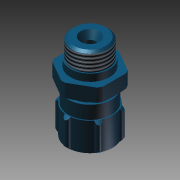
# Autodesk Inventor part: 2027 CK-1/8-PK-4
Saved by Autodesk Inventor 2016 (Build 200138000, 138)
## iProperties
Category: PARTsolutions
Company: FESTO
Created: 2018-04-08
Part Number: 2027 CK-1/8-PK-4
Catalog Web Link: www.cadenas.de
Description: CK-Quick connector
Vendor: FESTO
Document SubType Name: Modeling
Designer: psAdmin
Manufacturer: FESTO
Mass: 2.07705 g
Surface Area: 16.8691 cm^2
Volume: 2.07705 cm^3
Density: 1 g/cm^3
Material: Generic
Appearance: PSOLRGB-0-145-219
PSOL_IDENT_0: {$CADENAS_DATA\23d-libs\festo\parts\c\ck\ck.prj},170 {VTYP=3D},{NB=2027 CK-1/8-PK-4},{LINA=2027 CK-1
PSOL_IDENT_1: /8-PK-4},{NN=CK},{DATE=02.09.2015 08:31:43},{GEOMDATE=02.09.2015 08:31:43},{VERSION=},{LINEID=40},{L
PSOL_IDENT_2: INESUBID=-1},{WBVAR=}  {NB=2027 CK-1/8-PK-4},{LINA=2027 CK-1/8-PK-4},{KT=4},{TNR=2027},{TYP=CK-1/8-P
PSOL_IDENT_3: K-4},{A=24.700},{B=4.900},{C=G1/8A},{SW1=13.000},{SW2=12.000},{NW=2.900},{AD=4.000},{MB=3.700},{DK=1
PSOL_IDENT_4: 4.200},{NDR=9.728},{KDR=8.566},{TYP1=4.000}
NN: CK
NT: Quick connector
NB: 2027 CK-1/8-PK-4
NBSYN: $TNR. $TYP.
LINA: 2027 CK-1/8-PK-4
TNR: 2027
TYP: CK-1/8-PK-4
A: 24.700
B: 4.900
C: G1/8A
SW1: 13.000
SW2: 12.000
NW: 2.900
AD: 4.000
SUPPLIER: FESTO
ARTICLENO: 2027 CK-1/8-PK-4
BOMINFO: 2027 CK-1/8-PK-4
CREATOR: CADENAS GmbH
Title: 2027 CK-1/8-PK-4
Author: Cadenas PARTsolutions
Comments: Quick connector
Autodesk Inventor part; units mm, degrees
sketch "Sketch_1" plane through (0, 0, 0) normal (1, 0, 0) x (0, 1, 0)
  line L0 (0, -22.7) -> (0, -11.7)
  line L1 (0, -11.7) -> (5.75, -11.7)
  line L2 (5.75, -11.7) -> (5.75, -22.7)
  line L3 (5.75, -22.7) -> (0, -22.7)
  line L4 (0, -22.7) -> (0, -11.7)
  constraints: 10 end point
revolve "Revolution1" add sketch "Sketch_1" angle 360 about axis through (0, 0, -22.7) along (0, 0, -1)
sketch "Sketch_2" plane through (0, 0, 0) normal (1, 0, 0) x (0, 1, 0)
  line L0 (0, -22.7) -> (0, -11.7)
  line L1 (0, -11.7) -> (5, -11.7)
  line L2 (5, -11.7) -> (4.4585, -12.2415)
  line L3 (4.4585, -12.2415) -> (4.4585, -20.7)
  line L4 (4.4585, -20.7) -> (3.1, -22.0585)
  line L5 (3.1, -22.0585) -> (3.1, -22.7)
  line L6 (3.1, -22.7) -> (0, -22.7)
  line L7 (0, -22.7) -> (0, -11.7)
  constraints: 16 end point
revolve "Revolution2" cut sketch "Sketch_2" angle 360 about axis through (0, 0, -22.7) along (0, 0, -1)
thread "Thread1" size "M10x1" class "6H" standard "ISO Metric profile" length 5.9585
sketch "Sketch_3" plane through (0, 0, -15.2) normal (0, 0, 1) x (1, 0, 0)
  arc A0 (-5.5298, 2.3283) -> (-5.5298, -2.3283) centre (0, 0) ccw
  arc A1 (-5.5298, -2.3283) -> (-4.7813, -3.6248) centre (-5.1962, -3) ccw
  arc A2 (-4.7813, -3.6248) -> (-0.7485, -5.9531) centre (0, 0) ccw
  arc A3 (-0.7485, -5.9531) -> (0.7485, -5.9531) centre (0, -6) ccw
  arc A4 (0.7485, -5.9531) -> (4.7813, -3.6248) centre (0, 0) ccw
  arc A5 (4.7813, -3.6248) -> (5.5298, -2.3283) centre (5.1962, -3) ccw
  arc A6 (5.5298, -2.3283) -> (5.5298, 2.3283) centre (0, 0) ccw
  arc A7 (5.5298, 2.3283) -> (4.7813, 3.6248) centre (5.1962, 3) ccw
  arc A8 (4.7813, 3.6248) -> (0.7485, 5.9531) centre (0, 0) ccw
  arc A9 (0.7485, 5.9531) -> (-0.7485, 5.9531) centre (0, 6) ccw
  arc A10 (-0.7485, 5.9531) -> (-4.7813, 3.6248) centre (0, 0) ccw
  arc A11 (-4.7813, 3.6248) -> (-5.5298, 2.3283) centre (-5.1962, 3) ccw
  circle A12 centre (0, 0) radius 5.175
  constraints: 24 point on circle, 13 centre point
extrude "Extrusion1" add sketch "Sketch_3" against normal blind 7.5
sketch "Sketch_4" plane through (0, 0, 0) normal (1, 0, 0) x (0, 1, 0)
  line L0 (0, -23.7) -> (0, -14.2)
  line L1 (17.5375, -14.2) -> (6.0375, -14.2)
  line L2 (6.0375, -14.2) -> (6.0375, -15.2)
  line L3 (6.0375, -15.2) -> (9.7875, -18.95)
  line L4 (9.7875, -18.95) -> (5.0375, -23.7)
  line L5 (5.0375, -23.7) -> (17.5375, -23.7)
  line L6 (17.5375, -23.7) -> (17.5375, -14.2)
  constraints: 14 end point
revolve "Revolution3" cut sketch "Sketch_4" angle 360 about axis through (0, 0, -23.7) along (0, 0, -1)
sketch "Sketch_5" plane through (0, 0, 0) normal (1, 0, 0) x (0, 1, 0)
  line L0 (0, -24.7) -> (0, 0)
  line L1 (0, 0) -> (4.283, 0)
  line L2 (4.283, 0) -> (4.864, -0.581)
  line L3 (4.864, -0.581) -> (4.864, -4.9)
  line L4 (4.864, -4.9) -> (5.2, -4.9)
  line L5 (5.2, -4.9) -> (5.2, -6.8)
  line L6 (5.2, -6.8) -> (7.2, -6.8)
  line L7 (7.2, -6.8) -> (7.2, -10.3124)
  line L8 (7.2, -10.3124) -> (6.5, -10.5)
  line L9 (6.5, -10.5) -> (5.4, -10.5)
  arc A0 (5.4, -10.5) -> (5, -10.9) centre (5.4, -10.9) ccw
  line L10 (5, -10.9) -> (5, -17.1)
  line L11 (5, -17.1) -> (4.4, -17.7)
  line L12 (4.4, -17.7) -> (2.6, -17.7)
  arc A1 (2.6, -17.7) -> (2.4, -17.9) centre (2.6, -17.9) ccw
  line L13 (2.4, -17.9) -> (2.4, -21.5)
  arc A2 (2.5976, -21.8207) -> (2.4, -21.5) centre (2.3, -21.7828) ccw
  line L14 (2.5976, -21.8207) -> (1.95, -23.6)
  line L15 (1.95, -23.6) -> (1.95, -24.4)
  arc A3 (1.65, -24.7) -> (1.95, -24.4) centre (1.65, -24.4) ccw
  line L16 (1.65, -24.7) -> (0, -24.7)
  line L17 (0, -24.7) -> (0, 0)
  constraints: 36 end point, 8 point on circle, 4 centre point
revolve "Revolution4" add sketch "Sketch_5" angle 360 about axis through (0, 0, -24.7) along (0, 0, -1)
thread "Thread2" size "G9.728x0.907" designation "G 1/8" class "A" standard "ISO Pipe Threads" full length
sketch "Sketch_6" plane through (0, 0, -10.5) normal (0, 0, 1) x (1, 0, 0)
  line L0 (-13, -13) -> (13, -13)
  line L1 (13, -13) -> (13, 13)
  line L2 (13, 13) -> (-13, 13)
  line L3 (-13, 13) -> (-13, -13)
  line L4 (-6.5, 3.7528) -> (-6.5, -3.7528)
  line L5 (-6.5, -3.7528) -> (0, -7.5056)
  line L6 (0, -7.5056) -> (6.5, -3.7528)
  line L7 (6.5, -3.7528) -> (6.5, 3.7528)
  line L8 (6.5, 3.7528) -> (0, 7.5056)
  line L9 (0, 7.5056) -> (-6.5, 3.7528)
  constraints: 20 end point
extrude "Extrusion2" cut sketch "Sketch_6" along normal blind 3.7
sketch "Sketch_7_ALT_Drilling_1" plane through (0, 0, 0) normal (1, 0, 0) x (0, 1, 0)
  line L0 (0, -24.7) -> (0, 0)
  line L1 (0, 0) -> (2.4892, 0)
  line L2 (2.4892, 0) -> (1.45, -1.8)
  line L3 (1.45, -1.8) -> (1.45, -24.7)
  line L4 (1.45, -24.7) -> (0, -24.7)
  line L5 (0, -24.7) -> (0, 0)
  constraints: 12 end point
revolve "Revolution5" cut sketch "Sketch_7_ALT_Drilling_1" angle 360 about axis through (0, 0, -24.7) along (0, 0, -1)
ref_plane "ANBAU_XY" through (0, 0, -4.9) normal (0, 0, 1) x (1, 0, 0)
ref_plane "ANBAU_YZ" through (0, 0, -4.9) normal (1, 0, 0) x (0, 1, 0)
ref_plane "ANBAU_ZX" through (0, 0, -4.9) normal (0, 1, 0) x (0, 0, 1)
body "Solid1"
